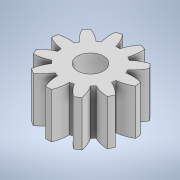
# Autodesk Inventor part: motor gear
Saved by Autodesk Inventor 2022 (Build 260153000, 153)
## iProperties
Created: 2024-01-22
Part Number: motor gear
Material: Типовые
Document SubType Name: Modeling
Designer: akapu
Density: 1 g/cm^3
Appearance: По умолчанию
Author: akapu
Autodesk Inventor part; units mm, degrees
ref_plane "YZ Plane" through (0, 0, 0) normal (1, 0, 0) x (0, 1, 0)
ref_plane "XZ Plane" through (0, 0, 0) normal (0, 1, 0) x (-1, 0, 0)
ref_plane "XY Plane" through (0, 0, 0) normal (0, 0, 1) x (1, 0, 0)
sketch "Эскиз1" plane through (0, 0, 0) normal (0, 1, 0) x (-1, 0, 0)
  circle A0 centre (0, 0) radius 2
  arc A1 (-3.8953, 5.2035) -> (-3.0052, 3.0052) centre (1.8465, 6.249) ccw
  arc A2 (-3.0052, 3.0052) -> (-3.4023, 2.5469) centre (0, 0) ccw
  arc A3 (-3.4023, 2.5469) -> (-5.7049, 3.1151) centre (-5.9226, -2.7171) ccw
  arc A4 (-5.7049, 3.1151) -> (-6.0902, 2.2715) centre (0, 0) ccw
  arc A5 (-6.0902, 2.2715) -> (-4.1529, 0.9034) centre (-1.8251, 6.2553) ccw
  arc A6 (-4.1529, 0.9034) -> (-4.2392, 0.3032) centre (0, 0) ccw
  arc A7 (-4.2392, 0.3032) -> (-6.4834, -0.4637) centre (-3.5135, -5.4878) ccw
  arc A8 (-6.4834, -0.4637) -> (-6.3515, -1.3817) centre (0, 0) ccw
  arc A9 (-6.3515, -1.3817) -> (-3.982, -1.4852) centre (-4.9172, 4.2756) ccw
  arc A10 (-3.982, -1.4852) -> (-3.7301, -2.0368) centre (0, 0) ccw
  arc A11 (-3.7301, -2.0368) -> (-5.2035, -3.8953) centre (0.0112, -6.5161) ccw
  arc A12 (-5.2035, -3.8953) -> (-4.5962, -4.5962) centre (0, 0) ccw
  arc A13 (-4.5962, -4.5962) -> (-2.5469, -3.4023) centre (-6.4482, 0.9384) ccw
  arc A14 (-2.5469, -3.4023) -> (-2.0368, -3.7301) centre (0, 0) ccw
  arc A15 (-2.0368, -3.7301) -> (-2.2715, -6.0902) centre (3.5323, -5.4757) ccw
  arc A16 (-2.2715, -6.0902) -> (-1.3817, -6.3515) centre (0, 0) ccw
  arc A17 (-1.3817, -6.3515) -> (-0.3032, -4.2392) centre (-5.9319, -2.6967) ccw
  arc A18 (-0.3032, -4.2392) -> (0.3032, -4.2392) centre (0, 0) ccw
  arc A19 (0.3032, -4.2392) -> (1.3817, -6.3515) centre (5.9319, -2.6967) ccw
  arc A20 (1.3817, -6.3515) -> (2.2715, -6.0902) centre (0, 0) ccw
  arc A21 (2.2715, -6.0902) -> (2.0368, -3.7301) centre (-3.5323, -5.4757) ccw
  arc A22 (2.0368, -3.7301) -> (2.5469, -3.4023) centre (0, 0) ccw
  arc A23 (2.5469, -3.4023) -> (4.5962, -4.5962) centre (6.4482, 0.9384) ccw
  arc A24 (4.5962, -4.5962) -> (5.2035, -3.8953) centre (0, 0) ccw
  arc A25 (5.2035, -3.8953) -> (3.7301, -2.0368) centre (-0.0112, -6.5161) ccw
  arc A26 (3.7301, -2.0368) -> (3.982, -1.4852) centre (0, 0) ccw
  arc A27 (3.982, -1.4852) -> (6.3515, -1.3817) centre (4.9172, 4.2756) ccw
  arc A28 (6.3515, -1.3817) -> (6.4834, -0.4637) centre (0, 0) ccw
  arc A29 (6.4834, -0.4637) -> (4.2392, 0.3032) centre (3.5135, -5.4878) ccw
  arc A30 (4.2392, 0.3032) -> (4.1529, 0.9034) centre (0, 0) ccw
  arc A31 (4.1529, 0.9034) -> (6.0902, 2.2715) centre (1.8251, 6.2553) ccw
  arc A32 (6.0902, 2.2715) -> (5.7049, 3.1151) centre (0, 0) ccw
  arc A33 (5.7049, 3.1151) -> (3.4023, 2.5469) centre (5.9226, -2.7171) ccw
  arc A34 (3.4023, 2.5469) -> (3.0052, 3.0052) centre (0, 0) ccw
  arc A35 (3.0052, 3.0052) -> (3.8953, 5.2035) centre (-1.8465, 6.249) ccw
  arc A36 (3.8953, 5.2035) -> (3.1151, 5.7049) centre (0, 0) ccw
  arc A37 (3.1151, 5.7049) -> (1.4852, 3.982) centre (6.4514, 0.9163) ccw
  arc A38 (1.4852, 3.982) -> (0.9034, 4.1529) centre (0, 0) ccw
  arc A39 (0.9034, 4.1529) -> (0.4637, 6.4834) centre (-4.9319, 4.2587) ccw
  arc A40 (0.4637, 6.4834) -> (-0.4637, 6.4834) centre (0, 0) ccw
  arc A41 (-0.4637, 6.4834) -> (-0.9034, 4.1529) centre (4.9319, 4.2587) ccw
  arc A42 (-0.9034, 4.1529) -> (-1.4852, 3.982) centre (0, 0) ccw
  arc A43 (-1.4852, 3.982) -> (-3.1151, 5.7049) centre (-6.4514, 0.9163) ccw
  arc A44 (-3.1151, 5.7049) -> (-3.8953, 5.2035) centre (0, 0) ccw
  constraints: 88 point on circle, 45 centre point
extrude "Выдавливание1" add sketch "Эскиз1" along normal blind 7
